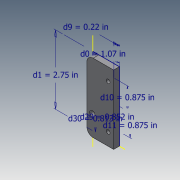
# Autodesk Inventor part: VP SWITCHMNT C
Saved by Autodesk Inventor 2018.3 (Build 223284000, 284)
## iProperties
Created: 2020-01-27
Material: Generic
Vendor: HHMI: JRC - ID&F
Document SubType Name: Modeling
Designer: arnoldj
Density: 1 g/cm^3
Appearance: Default
RuleStatus: InUse
AfterDocSave0: file://Part Number Cleaner
DESIGN DEPARTMENT: HHMI: JRC - ID&F
ALTERED ITEM PART NUMBER: N/A
ALTERED ITEM VENDOR: N/A
ALTERED ITEM DESCRIPTION: N/A
Author: arnoldj
Revision Number: 0
Autodesk Inventor part; units mm, degrees
ref_plane "YZ Plane" through (0, 0, 0) normal (1, 0, 0) x (0, 1, 0)
ref_plane "XZ Plane" through (0, 0, 0) normal (0, 1, 0) x (-1, 0, 0)
ref_plane "XY Plane" through (0, 0, 0) normal (0, 0, 1) x (1, 0, 0)
sketch "Sketch1" plane through (0, 0, 0) normal (0, 0, 1) x (1, 0, 0)
  line L0 (0, 83.82) -> (0, -13.97) projected
  line L1 (-5.4356, 0) -> (32.6136, 0) projected
  line L2 (0, 0) -> (27.178, 0)
  line L3 (27.178, 0) -> (27.178, 69.85)
  line L4 (27.178, 69.85) -> (0, 69.85)
  line L5 (0, 69.85) -> (0, 0)
  line L6 (0, 34.925) -> (27.178, 34.925) construction
  point P0 (5.5372, 20.6502)
  point P1 (21.59, 57.15)
  point P2 (21.59, 12.7)
  dimension "d0" = 27.178
  dimension "d1" = 69.85
  dimension "d9" = 5.588
  dimension "d10" = 22.225
  dimension "d11" = 22.225
  dimension "d29" = 21.6408
  dimension "d30" = 20.6502
  constraints: 10 end point, 2 midpoint, 2 parallel, 1 horizontal, 1 perpendicular, 1 vertical alignment
  measures "d0" distance of L3.end L4.end
  measures "d1" distance of L4.end L2.start
  measures "d9" distance from line of point (21.59, 57.15) L3
  measures "d10" distance from line of point (21.59, 57.15) L6
  measures "d11" distance from line of L6 point (21.59, 12.7)
  measures "d29" distance from line of L3 point (5.537, 20.65)
  measures "d30" distance from line of point (5.537, 20.65) L1
extrude "Extrusion1" add sketch "Sketch1" along normal blind 5.842
hole "Hole1" at (21.59, 57.15, 0) at (21.59, 12.7, 0) direction (0, 0, 1) diameter 3.81 end through all
hole "Hole2" at (5.5372, 20.6502, 0) direction (0, 0, 1) diameter 5.3594 end through all clearance for "Flat Head Machine Screw (82)" size "#10" standard "Ansi Unified Screw Threads"
fillet "Fillet1" radius 6.35 2 edges at (0, 69.85, 2.921) (0, 0, 2.921)
body "Solid1"
